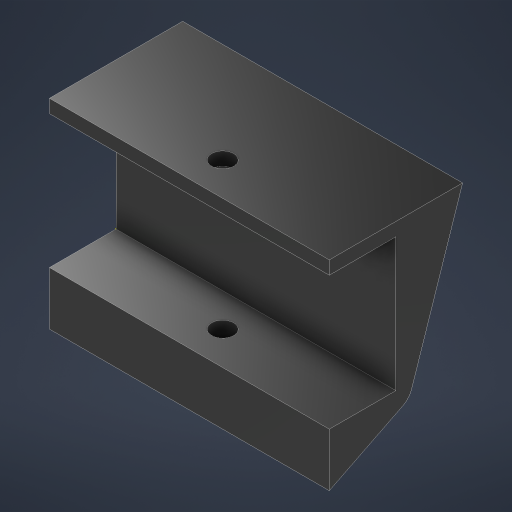
# Autodesk Inventor part: sleds v1
Saved by Autodesk Inventor 2024 (Build 280153000, 153)
## iProperties
Created: 2023-12-19
Part Number: sleds v1
Material: Generic
Document SubType Name: Modeling
Designer: elite
Density: 1 g/cm^3
Appearance: Glossy - Black
Author: elite
Autodesk Inventor part; units mm, degrees
ref_plane "YZ Plane" through (0, 0, 0) normal (1, 0, 0) x (0, 1, 0)
ref_plane "XZ Plane" through (0, 0, 0) normal (0, 1, 0) x (-1, 0, 0)
ref_plane "XY Plane" through (0, 0, 0) normal (0, 0, 1) x (1, 0, 0)
sketch "Sketch1" plane through (0, 0, 0) normal (1, 0, 0) x (0, 1, 0)
  line L0 (0, 0) -> (25.4, 0)
  line L1 (25.4, 0) -> (25.4, 12.7)
  line L2 (0, 0) -> (0, 12.7)
  line L3 (25.4, 12.7) -> (27.9305, 12.7)
  line L4 (27.9305, 12.7) -> (27.9305, 0)
  line L5 (0, 12.7) -> (-2.54, 12.7)
  line L6 (-2.54, 12.7) -> (-2.54, 0)
  line L7 (-2.54, 0) -> (-2.54, -2.54)
  line L8 (27.9305, -2.54) -> (27.9305, 0)
  line L9 (-2.54, -2.54) -> (-2.54, -12.7002)
  line L10 (27.9305, -12.7002) -> (27.9305, -2.54)
  line L11 (27.9305, -12.7002) -> (-2.54, -2.54)
  line L12 (-2.54, 12.7) -> (-10.16, 12.7)
  line L13 (-10.16, 12.7) -> (-2.54, -2.54)
  line L14 (-2.54, -2.54) -> (0, -2.54)
  dimension "d0" = 25.4
  dimension "d1" = 12.7
  dimension "d2" = 2.54
  dimension "d3" = 2.54
  dimension "d4" = 7.62
  constraints: 30 end point, 4 horizontal, 4 perpendicular, 3 point on line, 3 vertical
  measures "d0" distance of L0.start L0.end
  measures "d1" distance of L0.end L1.end
  measures "d2" distance of L2.end L5.end
  measures "d3" distance of L6.end L7.end
  measures "d4" distance of L5.end L12.end
extrude "Extrusion1" add sketch "Sketch1" along normal blind 53.34
sketch "Sketch2" plane through (0, 27.9305, 12.7) normal (0, 1, 0) x (1, 0, 0)
  line L0 (0, 0) -> (0, 12.7) projected
  line L1 (0, 0) -> (0, 6.35)
  line L2 (0, 6.35) -> (26.67, 6.35)
  circle A0 centre (26.67, 6.35) radius 2.1082
  dimension "d7" = 6.35
  dimension "d8" = 26.67
  dimension "d9" = 4.2164
  constraints: 4 end point, 1 centre point, 1 coincident, 1 midpoint, 1 perpendicular
  measures "d7" distance of L0.start L1.end
  measures "d8" distance of L1.end L2.end
  measures "d9" diameter of A0
extrude "Extrusion2" cut sketch "Sketch2" against normal blind 54.61
sketch "Sketch3" plane through (0, 0, 0) normal (-1, 0, 0) x (0, 0, 1)
  point P0 (0, 0)
sketch "Sketch4" plane through (0, 0, 12.7) normal (0, 1, 0) x (1, 0, 0)
  circle A0 centre (26.67, 6.35) radius 2.1082 projected
  circle A1 centre (26.67, 6.35) radius 2.1082
  circle A2 centre (26.67, 6.35) radius 5.0752
  point P0 (0, 12.7)
  constraints: 2 centre point, 2 coincident
extrude "Extrusion3" cut sketch "Sketch4" against normal up to surface from surface at 0 surface through (0, -10.16, 12.7) normal (0, -0.8944, -0.4472)
sketch "Sketch5" plane through (0, 0, 12.7) normal (0, 1, 0) x (1, 0, 0)
  circle A0 centre (26.67, 6.35) radius 5.0752 projected
  circle A1 centre (26.67, 6.35) radius 5.0752
  circle A2 centre (26.67, 6.35) radius 2.1082
  point P0 (0, 12.7)
  dimension "d14" = 4.2164
  constraints: 2 centre point, 2 coincident
  measures "d14" diameter of A2
extrude "Extrusion4" add sketch "Sketch5" against normal blind 3.175
fillet "Fillet1" radius 3.175 1 edges at (26.67, -2.54, -2.54)
body "Solid1"
